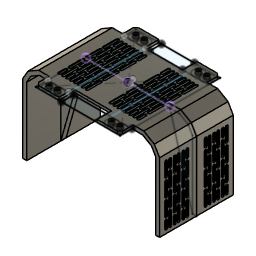
Suspension Electronics Cover (Autodesk Fusion 360 design; units mm, degrees)
Autodesk Fusion 360 part; units mm, degrees
sketch "Sketch1" plane through (0, 0, 0) normal (0, 0, 1) x (1, 0, 0)
  line L0 (32, 38) -> (-32, 38)
  line L1 (-32, 38) -> (-32, -38)
  line L2 (-32, -38) -> (32, -38)
  line L3 (32, -38) -> (32, 38)
  line L4 (32, 38) -> (-32, -38) construction
  line L5 (-32, 38) -> (32, -38) construction
  line L6 (0, 0) -> (0, 3.6901)
  line L7 (0, 0) -> (2, 0)
  circle A0 centre (-20.55, 33) radius 1.7
  circle A1 centre (20.55, 33) radius 1.7
  circle A2 centre (-27, -33) radius 1.7
  circle A3 centre (27, -33) radius 1.7
  circle A4 centre (-27, 33) radius 1.7
  circle A5 centre (27, 33) radius 1.7
  line L8 (-32, 29) -> (32, 29)
  line L9 (-32, -29) -> (32, -29)
  circle A6 centre (-20.55, -33) radius 1.7
  circle A7 centre (20.55, -33) radius 1.7
  circle A8 centre (-27, -33) radius 4
  circle A9 centre (-20.55, -33) radius 4
  circle A10 centre (20.55, -33) radius 4
  circle A11 centre (27, -33) radius 4
  circle A12 centre (20.55, 33) radius 4
  circle A13 centre (27, 33) radius 4
  circle A14 centre (-27, 33) radius 4
  circle A15 centre (-20.55, 33) radius 4
  line L10 (12.5, -38) -> (12.5, -29)
  line L11 (-12.5, -38) -> (-12.5, -29)
  line L12 (12.5, 38) -> (12.5, 29)
  line L13 (-12.5, 38) -> (-12.5, 29)
  line L14 (16, -29) -> (16, 29)
  line L15 (-16, -29) -> (-16, 29)
  dimension "d1" = 76
  dimension "d4" = 20.55
  dimension "d5" = 33
  dimension "d6" = 64
  dimension "d7" = 3.4
  dimension "d8" = 33
  dimension "d9" = 54
  dimension "d41" = 9
  dimension "d47" = 8
  dimension "d52" = 25
  constraint horizontal L0
  constraint perpendicular L0 L1
  constraint parallel L0 L2
  constraint parallel L1 L3
  constraint coincident L4 L6.start
  constraint coincident L5 L6.start
  constraint coincident L6.start L7.start
  constraint vertical L6
  constraint perpendicular L6 L7
  constraint symmetric L6 A0 A1
  constraint equal A0 A2
  constraint symmetric L6 A2 A3
  constraint symmetric L7 A2 A4
  constraint symmetric L7 A3 A5
  constraint coincident L3 L8.end
  constraint perpendicular L3 L8
  constraint symmetric L7 L8.start L9.start
  constraint symmetric L7 L8.end L9.end
  constraint symmetric L7 A0 A6
  constraint symmetric L7 A1 A7
  constraint concentric A2 A8
  constraint concentric A6 A9
  constraint concentric A7 A10
  constraint concentric A3 A11
  constraint concentric A1 A12
  constraint concentric A5 A13
  constraint concentric A4 A14
  constraint concentric A0 A15
  constraint equal A8 A9
  constraint equal A9 A10
  constraint equal A10 A11
  constraint equal A11 A13
  constraint equal A12 A13
  constraint equal A12 A15
  constraint equal A14 A15
  constraint coincident L2 L10.start
  constraint coincident L9 L10.end
  constraint perpendicular L9 L10
  constraint symmetric L6 L10.start L11.start
  constraint symmetric L6 L10.end L11.end
  constraint symmetric L7 L10.start L12.start
  constraint symmetric L7 L10.end L12.end
  constraint symmetric L7 L11.start L13.start
  constraint symmetric L7 L11.end L13.end
  constraint coincident L9 L14.start
  constraint coincident L8 L14.end
  constraint perpendicular L8 L14
  constraint symmetric L6 L14.start L15.start
  constraint symmetric L6 L14.end L15.end
  measures "d1" distance of L0.end L1.end
  measures "d4" distance of L6 A0.centre
  measures "d5" vertical distance of L6.start A0.centre
  measures "d6" distance of L1 L3
  measures "d7" diameter of A0
  measures "d8" vertical distance of L6.start A2.centre
  measures "d9" distance of A2.centre A3.centre
  measures "d41" distance of L0 L8
  measures "d47" diameter of A8
  measures "d52" distance of L10 L11
extrude "Extrude1" add sketch "Sketch1" along normal blind 2 contours L0 L3 L8 A12 A13 L12 | L3 L8 L9 L14 | L0 L1 L8 A14 A15 L13 | L8 L9 L14 L15 | L2 L3 L9 A10 A11 L10 | L8 A12 A13 | A12 A13 | L9 A10 A11 | A10 A11 | A12 A13 | A12 A13 | L1 L8 L9 L15 | A10 A11 | A10 A11 | L1 L2 L9 A8 A9 L11 | L8 A14 A15 | A14 A15 | A14 A15 | L9 A8 A9 | A8 A9 | A14 A15 | A8 A9 | A8 A9
extrude "Extrude3" [suppressed]
chamfer "Chamfer1" distance 2 angle 45 4 edges at (-32, -38, 1) (32, -38, 1) (-32, 38, 1) (32, 38, 1)
sketch "Sketch2" plane through (0, 0, 2) normal (0, 0, 1) x (-1, 0, 0)
  line L0 (-32, -36) -> (-30, -38)
  line L1 (-30, -38) -> (-12.5, -38)
  line L2 (30, -38) -> (32, -36)
  line L3 (32, -36) -> (32, 36)
  line L4 (32, 36) -> (30, 38)
  line L5 (30, 38) -> (12.5, 38)
  line L6 (-30, 38) -> (-32, 36)
  line L7 (-32, 36) -> (-32, -36)
  circle A0 centre (20.55, -33) radius 1.7
  circle A1 centre (27, 33) radius 1.7
  circle A2 centre (-27, 33) radius 1.7
  circle A3 centre (-20.55, -33) radius 1.7
  line L8 (31, -22) -> (31, -12)
  arc A4 (31, -12) -> (29, -12) centre (30, -12) ccw
  line L9 (29, -12) -> (29, -22)
  arc A5 (29, -22) -> (31, -22) centre (30, -22) ccw
  line L10 (30, -22) -> (30, -12) construction
  line L11 (31, -9) -> (31, -4)
  arc A6 (31, -4) -> (29, -4) centre (30, -4) ccw
  line L12 (29, -4) -> (29, -9)
  arc A7 (29, -9) -> (31, -9) centre (30, -9) ccw
  line L13 (30, -9) -> (30, -4) construction
  line L14 (28, -22) -> (28, -17)
  arc A8 (28, -17) -> (26, -17) centre (27, -17) ccw
  line L15 (26, -17) -> (26, -22)
  arc A9 (26, -22) -> (28, -22) centre (27, -22) ccw
  line L16 (27, -22) -> (27, -17) construction
  line L17 (28, -14) -> (28, -4)
  arc A10 (28, -4) -> (26, -4) centre (27, -4) ccw
  line L18 (26, -4) -> (26, -14)
  arc A11 (26, -14) -> (28, -14) centre (27, -14) ccw
  line L19 (27, -14) -> (27, -4) construction
  line L20 (30, -22) -> (29.6, -22)
  circle A12 centre (-27, -33) radius 1.7
  circle A13 centre (27, -33) radius 1.7
  circle A14 centre (-20.55, 33) radius 1.7
  circle A15 centre (20.55, 33) radius 1.7
  line L21 (-12.5, -38) -> (-12.5, -29)
  line L22 (-12.5, -29) -> (12.5, -29)
  line L23 (12.5, -29) -> (12.5, -38)
  line L24 (12.5, 38) -> (12.5, 29)
  line L25 (12.5, 29) -> (-12.5, 29)
  line L26 (-12.5, 29) -> (-12.5, 38)
  line L27 (12.5, -38) -> (30, -38)
  line L28 (-12.5, 38) -> (-30, 38)
  dimension "d13" = 2
  dimension "d14" = 10
  dimension "d15" = 2
  dimension "d16" = 16
  dimension "d24" = 2
  dimension "d25" = 5
  dimension "d26" = 3
  dimension "d27" = 2
  dimension "d28" = 2
  dimension "d29" = 3
  dimension "d30" = 5
  dimension "d31" = 10
  dimension "d32" = 3
  constraint tangent L8 A4
  constraint tangent A4 L9
  constraint parallel L8 L9
  constraint tangent L9 A5
  constraint tangent L8 A5
  constraint vertical L10
  constraint tangent L11 A6
  constraint tangent A6 L12
  constraint parallel L11 L12
  constraint tangent L12 A7
  constraint tangent L11 A7
  constraint vertical L13
  constraint collinear A5.centre A4.centre A7.centre
  constraint tangent L14 A8
  constraint tangent A8 L15
  constraint parallel L14 L15
  constraint tangent L15 A9
  constraint tangent L14 A9
  constraint vertical L16
  constraint tangent L17 A10
  constraint tangent A10 L18
  constraint parallel L17 L18
  constraint tangent L18 A11
  constraint tangent L17 A11
  constraint parallel L15 L19
  constraint coincident A5.centre L10.start
  constraint perpendicular L10 L20
  constraint collinear A5.centre A9.centre L20.end
  constraint collinear A9.centre A8.centre A11.centre
  measures "d13" diameter of A4
  measures "d14" distance of A5.centre A4.centre
  measures "d15" distance of L3 L10
  measures "d16" distance of L1 A5.centre
  measures "d24" diameter of A6
  measures "d25" distance of A7.centre A6.centre
  measures "d26" distance of A4.centre A7.centre
  measures "d27" diameter of A10
  measures "d28" distance of L14 L15
  measures "d29" distance of A5.centre A9.centre
  measures "d30" distance of A9.centre A8.centre
  measures "d31" distance of A11.centre A10.centre
  measures "d32" vertical distance of A8.centre A11.centre
extrude "Extrude2" cut sketch "Sketch2" against normal blind 0.5 contours L8 A4 L9 A5 | L11 A6 L12 A7 | L14 A8 L15 A9 | L17 A10 L18 A11
sketch "Sketch3" plane through (0, 0, 0) normal (0, 1, 0) x (1, 0, 0)
  line L0 (0, 0) -> (0, -2)
  line L1 (0, -2) -> (40, -2)
  line L2 (40, -2) -> (48, 2.6188)
  line L3 (48, 2.6188) -> (52, 9.547)
  line L4 (52, 9.547) -> (52, 62)
  line L5 (52, 62) -> (49, 62)
  line L6 (49, 62) -> (49, 10.3509)
  line L7 (49, 10.3509) -> (45.8038, 4.815)
  line L8 (45.8038, 4.815) -> (39.1962, 1)
  line L9 (39.1962, 1) -> (0, 1)
  line L10 (0, 1) -> (0, 0)
  line L11 (32, 0) -> (-32, 0)
  line L12 (32, 1) -> (49, 62)
  line L13 (32, 1) -> (32, -2)
  dimension "d56" = 3
  dimension "d57" = 3
  dimension "d58" = 3
  dimension "d59" = 3
  dimension "d60" = 40
  dimension "d61" = 48
  dimension "d62" = 52
  dimension "d63" = 150
  dimension "d64" = 150
  dimension "d65" = 62
  dimension "d66" = 2
  dimension "d70" = 20
  dimension "d73" = 32
  constraint coincident L0.start L10.end
  constraint vertical L0
  constraint perpendicular L0 L1
  constraint parallel L0 L4
  constraint perpendicular L4 L5
  constraint perpendicular L5 L6
  constraint parallel L3 L7
  constraint parallel L0 L10
  constraint parallel L1 L9
  constraint parallel L2 L8
  constraint coincident L9 L12.start
  constraint coincident L1 L13.end
  constraint perpendicular L1 L13
  measures "d56" distance of L1 L9
  measures "d57" distance of L2 L8
  measures "d58" distance of L3 L7
  measures "d59" distance of L4 L6
  measures "d60" distance of L0.end L1.end
  measures "d61" distance of L2.end L10
  measures "d62" distance of L0 L4
  measures "d63" angle of L8 L9
  measures "d64" angle of L7 L8
  measures "d65" distance of L5 L0.start
  measures "d66" distance of L1 L11
  measures "d70" distance of L4 L12.start
  measures "d73" distance of L0 L13
extrude "Extrude5" add sketch "Sketch3" along normal mid plane 56 contours L1 L2 L3 L4 L5 L6 L7 L8 L9 L13
extrude "Extrude7" add sketch "Sketch3" along normal mid plane 48 contours L9 L10 L11 L13
move_face "OffsetFaces1" offset -2 6 faces at (12.5, 35, 0.6667) (-4.1667, 29, 0.6667) (-12.5, 35, 0.6667) (-12.5, -35, 0.6667) (-4.1667, -29, 0.6667) (12.5, -35, 0.6667)
extrude "Extrude6" add sketch "Sketch3" along normal mid plane 4 contours L6 L7 L8 L9 L12
mirror "Mirror2" about plane through (0, 0, 0) normal (1, 0, 0) of "Extrude5", "Extrude7", "Extrude6"
pattern_linear "R-Pattern1" count 4 spacing 6 along (1, 0, 0) count 3 spacing 13 along (0, -1, 0) of "Extrude2"
mirror "Mirror1" about plane through (0, 0, 0) normal (1, 0, 0) of "Extrude2", "R-Pattern1"
sketch "Sketch4" plane through (52, 0, 0) normal (1, 0, 0) x (0, 1, 0)
  line L0 (28, -9.547) -> (-28, -9.547)
  line L1 (-28, -9.547) -> (-28, -62)
  line L2 (-28, -62) -> (28, -62)
  line L3 (28, -62) -> (28, -9.547)
  line L4 (-21, -14.547) -> (-21, -19.547)
  line L5 (-24, -27.547) -> (-24, -32.547)
  line L6 (-20, -32.547) -> (-20.4, -32.547)
  line L7 (-24, -14.547) -> (-24, -24.547)
  line L8 (-23, -24.547) -> (-23, -14.547) construction
  arc A0 (-22, -14.547) -> (-24, -14.547) centre (-23, -14.547) ccw
  line L9 (-22, -32.547) -> (-22, -27.547)
  arc A1 (-21, -19.547) -> (-19, -19.547) centre (-20, -19.547) ccw
  arc A2 (-19, -22.547) -> (-21, -22.547) centre (-20, -22.547) ccw
  line L10 (-20, -32.547) -> (-20, -22.547) construction
  arc A3 (-22, -27.547) -> (-24, -27.547) centre (-23, -27.547) ccw
  line L11 (-21, -22.547) -> (-21, -32.547)
  line L12 (-20, -19.547) -> (-20, -14.547) construction
  line L13 (-22, -24.547) -> (-22, -14.547)
  arc A4 (-21, -32.547) -> (-19, -32.547) centre (-20, -32.547) ccw
  arc A5 (-19, -14.547) -> (-21, -14.547) centre (-20, -14.547) ccw
  arc A6 (-24, -32.547) -> (-22, -32.547) centre (-23, -32.547) ccw
  line L14 (-19, -32.547) -> (-19, -22.547)
  arc A7 (-24, -24.547) -> (-22, -24.547) centre (-23, -24.547) ccw
  line L15 (-23, -32.547) -> (-23, -27.547) construction
  line L16 (-19, -19.547) -> (-19, -14.547)
  dimension "d78" = 2
  dimension "d79" = 10
  dimension "d80" = 2
  dimension "d81" = 5
  dimension "d82" = 3
  dimension "d83" = 2
  dimension "d84" = 2
  dimension "d85" = 3
  dimension "d86" = 5
  dimension "d87" = 10
  dimension "d88" = 3
  dimension "d89" = 5
  dimension "d90" = 5
  constraint tangent A2 L14
  constraint tangent A2 L11
  constraint parallel L11 L14
  constraint tangent L11 A4
  constraint tangent A4 L14
  constraint vertical L10
  constraint tangent A5 L16
  constraint tangent L4 A5
  constraint parallel L4 L16
  constraint tangent L4 A1
  constraint tangent A1 L16
  constraint vertical L12
  constraint collinear A1.centre L6.start A2.centre
  constraint tangent L9 A3
  constraint tangent L5 A3
  constraint parallel L5 L9
  constraint tangent L5 A6
  constraint tangent L9 A6
  constraint vertical L15
  constraint tangent A0 L13
  constraint tangent L7 A0
  constraint parallel L7 L13
  constraint tangent L7 A7
  constraint tangent L13 A7
  constraint parallel L5 L8
  constraint coincident L6.start L10.start
  constraint perpendicular L6 L10
  constraint collinear L6.end A6.centre L6.start
  constraint collinear A3.centre A6.centre L8.start
  measures "d78" diameter of A2
  measures "d79" distance of L6.start A2.centre
  measures "d80" diameter of A5
  measures "d81" distance of A1.centre L12.end
  measures "d82" distance of A1.centre A2.centre
  measures "d83" diameter of A0
  measures "d84" distance of L5 L9
  measures "d85" distance of A6.centre L6.start
  measures "d86" distance of A3.centre A6.centre
  measures "d87" distance of L8.start L8.end
  measures "d88" vertical distance of A3.centre L8.start
  measures "d89" distance of L1 L8.end
  measures "d90" distance of L0 L8.end
extrude "Extrude8" cut sketch "Sketch4" against normal blind 1 contours L4 A1 A5 L16 | L5 L9 A3 A6 | L7 A0 L13 A7 | A2 L11 A4 L14
pattern_linear "R-Pattern2" count 3 spacing 13 along (0, 0, -1) count 3 spacing 6.5 along (0, 1, 0) of "Extrude8"
mirror "Mirror3" about plane through (0, 0, 0) normal (0, 1, 0) of "Extrude8", "R-Pattern2"
mirror "Mirror4" about plane through (0, 0, 0) normal (1, 0, 0) of "Extrude8", "R-Pattern2", "Mirror3"
equation "d1 = 66 mm + 10 mm"
equation "d4 = ( 41.1 / 2 ) * 1 mm"
equation "d5 = ( 66 / 2 ) * 1 mm"
equation "d74 = 28.00 mm - 4 mm"
